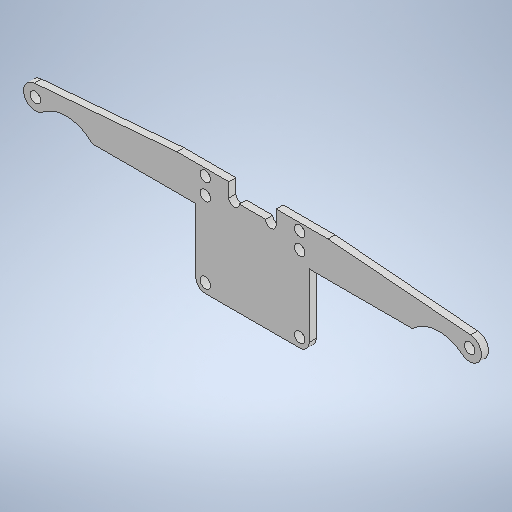
# Autodesk Inventor part: mata
Saved by Autodesk Inventor 2025.1 (Build 291241000, 241)
## iProperties
Created: 2024-08-31
Part Number: mata
Material: 一般
Document SubType Name: Modeling
Designer: right
Density: 1 g/cm^3
Appearance: 既定
Author: right
Autodesk Inventor part; units mm, degrees
ref_plane "YZ Plane" through (0, 0, 0) normal (1, 0, 0) x (0, 1, 0)
ref_plane "XZ Plane" through (0, 0, 0) normal (0, 1, 0) x (-1, 0, 0)
ref_plane "XY Plane" through (0, 0, 0) normal (0, 0, 1) x (1, 0, 0)
sketch "スケッチ1" plane through (0, 0, 0) normal (0, 0, 1) x (1, 0, 0)
  line L0 (-16, 5) -> (16, 5)
  circle A0 centre (-10, 0) radius 1.1
  line L1 (0, 5) -> (0, 0) construction
  circle A1 centre (10, 0) radius 1.1
  circle A2 centre (-10, -16) radius 1.1
  circle A3 centre (-46, 0) radius 1.1
  circle A4 centre (-46, 0) radius 2.5
  line L2 (-46.2069, 2.4914) -> (-16, 5)
  circle A5 centre (10, -16) radius 1.1
  circle A6 centre (46, 0) radius 1.1
  circle A7 centre (46, 0) radius 2.5
  line L3 (46.2069, 2.4914) -> (16, 5)
  circle A8 centre (-10, 0) radius 2
  circle A9 centre (-10, -16) radius 2
  circle A10 centre (10, -16) radius 2
  circle A11 centre (10, 0) radius 2
  line L4 (-10, -18) -> (10, -18)
  line L5 (-46, -2.5) -> (46, -2.5)
  line L6 (-12, 0) -> (-12, -16)
  line L7 (12, 0) -> (12, -16)
  circle A12 centre (-39.4996, -8) radius 10.308 construction
  circle A13 centre (-39.4996, -8) radius 7.808
  circle A14 centre (39.4996, -8) radius 7.808
  point P0 (-12, -8)
  point P1 (12, -2.5)
  point P2 (33.9575, -2.5)
  point P3 (44.4235, -1.9402)
  point P4 (-44.4235, -1.9402)
  point P5 (-33.9575, -2.5)
  point P6 (-12, -2.5)
  dimension "d9" = 4
  dimension "d12" = 4
  dimension "d13" = 20.616
  dimension "d0" = 2.2
  dimension "d1" = 5
  dimension "d2" = 20
  dimension "d4" = 2.2
  dimension "d5" = 16
  dimension "d6" = 2.2
  dimension "d7" = 36
  dimension "d8" = 5
  dimension "d10" = 4
  dimension "d11" = 4
  dimension "d32" = 30
  constraints: 16 end point, 12 centre point, 8 point on circle, 7 coincident, 7 tangent, 6 symmetric about line, 5 horizontal alignment, 3 vertical, 2 horizontal, 2 midpoint, 2 vertical alignment, 12 other
  measures "d0" diameter of A0
  measures "d1" distance from line of L0 A0.centre
  measures "d2" distance of A1.centre A0.centre
  measures "d4" diameter of A2
  measures "d5" distance of A2.centre A0.centre
  measures "d6" diameter of A3
  measures "d7" distance of A0.centre A3.centre
  measures "d8" diameter of A4
  measures "d10" diameter of A9
  measures "d11" diameter of A10
  measures "d32" horizontal distance of A3.centre L0.start
extrude "押し出し1" add sketch "スケッチ1" along normal blind 1.5 contours L0 L3 A7 A14 L5 A13 A4 L2 | A4 | A7 | L7 A10 L4 A9 L6 L5 | A10 | A9 | A8 | A11
sketch "スケッチ4" plane through (0, 0, 1.5) normal (0, 0, 1) x (1, 0, 0)
  line L0 (16, 5) -> (-16, 5) projected
  line L1 (-5, 5) -> (5, 5)
  line L2 (5, 5) -> (5, 2)
  line L3 (5, 2) -> (-5, 2)
  line L4 (-5, 2) -> (-5, 5)
  circle A0 centre (-3.9, 2) radius 1.1
  circle A1 centre (3.9, 2) radius 1.1
  circle A2 centre (-10, 3.5) radius 1.1
  line L5 (0, 5) -> (0, 2) construction
  circle A3 centre (10, 3.5) radius 1.1
  point P0 (0, 0)
  point P1 (-5, 3.5)
  point P2 (2.8, 2)
  point P3 (5, 5)
  point P4 (-2.8, 2)
  dimension "d26" = 2.2
  dimension "d27" = 2.2
  dimension "d24" = 10
  dimension "d25" = 3
  dimension "d28" = 2.2
  dimension "d29" = 5
  constraints: 10 end point, 3 midpoint, 3 point on line, 2 centre point, 2 parallel, 1 horizontal, 1 horizontal alignment, 1 perpendicular, 1 symmetric about line, 1 vertical, 1 vertical alignment, 7 other
  measures "d24" distance of L2.end L3.end
  measures "d25" distance between parallel lines of L0 L3
  measures "d28" diameter of A2
  measures "d29" distance from line of L4 A2.centre
extrude "押し出し4" cut sketch "スケッチ4" against normal through all
equation "\"d27\" = d26"
